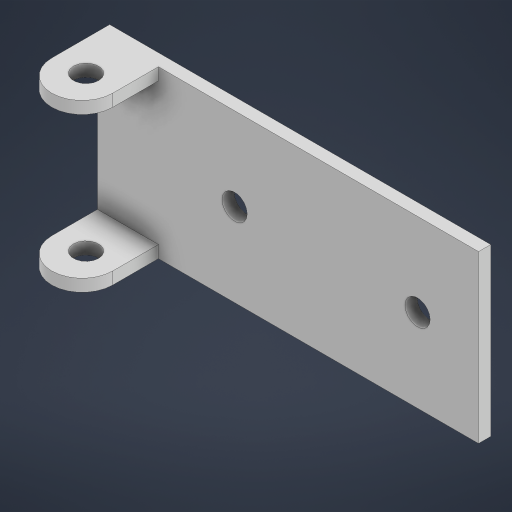
# Autodesk Inventor part: Base
Saved by Autodesk Inventor 2024.2 (Build 282272000, 272)
## iProperties
Created: 2024-06-05
Part Number: Base
Material: Generic
Document SubType Name: Modeling
Designer: simon
Density: 1 g/cm^3
Appearance: Default
Author: simon
Autodesk Inventor part; units mm, degrees
ref_plane "YZ Plane" through (0, 0, 0) normal (1, 0, 0) x (0, 1, 0)
ref_plane "XZ Plane" through (0, 0, 0) normal (0, 1, 0) x (-1, 0, 0)
ref_plane "XY Plane" through (0, 0, 0) normal (0, 0, 1) x (1, 0, 0)
sketch "Sketch1" plane through (0, 0, 0) normal (0, 0, 1) x (1, 0, 0)
  line L0 (0, 0) -> (50, 0)
  line L1 (50, 0) -> (50, 21.8)
  line L2 (50, 21.8) -> (0, 21.8)
  line L3 (0, 21.8) -> (0, 0)
  circle A0 centre (42, 10.9) radius 1.65
  circle A1 centre (18, 10.9) radius 1.65
  dimension "d0" = 50
  dimension "d1" = 21.8
  dimension "d15" = 3.3
  dimension "d16" = 3.3
  dimension "d17" = 24
  dimension "d18" = 8
  dimension "d19" = 10.9
  dimension "d20" = 10.9
  constraints: 8 end point, 2 centre point, 2 parallel, 1 horizontal, 1 perpendicular
  measures "d0" distance of L2.end L1.end
  measures "d1" distance of L1.end L0.end
  measures "d15" diameter of A0
  measures "d16" diameter of A1
  measures "d17" distance of A0.centre A1.centre
  measures "d18" distance from line of A0.centre L1
  measures "d19" distance from line of A0.centre L0
  measures "d20" distance from line of A1.centre L0
extrude "Extrusion1" add sketch "Sketch1" along normal blind 1.6
sketch "Sketch2" plane through (0, 0, 1.6) normal (0, 0, 1) x (1, 0, 0)
  line L0 (0, 21.8) -> (0, 0) projected
  line L1 (0, 0) -> (8, 0)
  line L2 (8, 0) -> (8, 1.6)
  line L3 (8, 1.6) -> (0, 1.6)
  line L4 (0, 1.6) -> (0, 0)
  line L5 (50, 21.8) -> (0, 21.8) projected
  line L6 (0, 21.8) -> (8, 21.8)
  line L7 (8, 21.8) -> (8, 20.2)
  line L8 (8, 20.2) -> (0, 20.2)
  line L9 (0, 20.2) -> (0, 21.8)
  point P0 (0, 20.2)
  dimension "d4" = 8
  dimension "d5" = 1.6
  dimension "d6" = 8
  dimension "d7" = 1.6
  constraints: 16 end point, 4 parallel, 2 horizontal, 2 perpendicular
  measures "d4" distance of L3.end L2.end
  measures "d5" distance of L2.end L1.end
  measures "d6" distance of L7.end L8.end
  measures "d7" distance of L6.end L7.end
extrude "Extrusion2" add sketch "Sketch2" along normal blind 10
sketch "Sketch3" plane through (0, 0, 0) normal (0, -1, 0) x (1, 0, 0)
  circle A0 centre (4, 7.1) radius 1.65
  line L0 (0, 0) -> (0, 11.6) projected
  line L1 (0, 11.6) -> (8, 11.6) projected
  line L2 (0, 0) -> (50, 0) projected
  dimension "d10" = 3.3
  dimension "d11" = 4
  dimension "d21" = 7.1
  constraints: 1 centre point
  measures "d10" diameter of A0
  measures "d11" distance from line of L0 A0.centre
  measures "d21" distance from line of A0.centre L2
extrude "Extrusion3" cut sketch "Sketch3" against normal blind 25
fillet "Fillet1" radius 4 4 edges at (8, 0.8, 11.6) (8, 21, 11.6) (0, 0.8, 11.6) (0, 21, 11.6)
body "Solid1"
